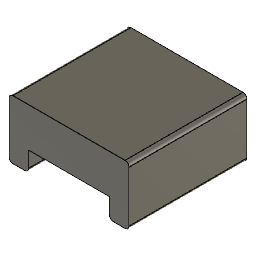
3) PLA 10mm Level Spacer (Autodesk Fusion 360 design; units mm, degrees)
Autodesk Fusion 360 part; units mm, degrees
sketch "Sketch1" plane through (0, 0, 0) normal (0, 0, 1) x (1, 0, 0)
  line L0 (10.25, 15) -> (-10.25, 15)
  line L1 (-10.25, 15) -> (-10.25, -15)
  line L2 (-10.25, -15) -> (10.25, -15)
  line L3 (10.25, -15) -> (10.25, 15)
  line L4 (10.25, 15) -> (-10.25, -15) construction
  line L5 (-10.25, 15) -> (10.25, -15) construction
  line L6 (-10.25, 15) -> (-15.25, 15)
  line L7 (-15.25, 15) -> (-15.25, -15)
  line L8 (-15.25, -15) -> (-10.25, -15)
  line L9 (-10.25, -15) -> (-10.25, 15)
  line L10 (10.25, 15) -> (15.25, 15)
  line L11 (15.25, 15) -> (15.25, -15)
  line L12 (15.25, -15) -> (10.25, -15)
  line L13 (10.25, -15) -> (10.25, 15)
  dimension "d1" = 20.5
  dimension "d2" = 30
  dimension "d3" = 5
  dimension "d4" = 30
  dimension "d5" = 5
  dimension "d6" = 30
  constraint horizontal L0
  constraint perpendicular L0 L1
  constraint parallel L0 L2
  constraint parallel L1 L3
  constraint coincident L4 origin
  constraint coincident L5 origin
  constraint horizontal L6
  constraint vertical L7
  constraint horizontal L8
  constraint vertical L9
  constraint horizontal L10
  constraint vertical L11
  constraint horizontal L12
  constraint vertical L13
  measures "d1" distance of L1.end L2.end
  measures "d2" distance of L0.end L1.end
  measures "d3" distance of L0.end L6.end
  measures "d4" distance of L0.end L1.end
  measures "d5" distance of L0.start L10.end
  measures "d6" distance of L0.start L2.end
extrude "Extrude1" add sketch "Sketch1" along normal blind 10
extrude "Extrude2" add sketch "Sketch1" against normal blind 5 contours L3 L10 L11 L12 L13 | L1 L6 L7 L8 L9
fillet "Fillet1" radius 1 6 edges at (-10.25, 0, -5) (10.25, 0, -5) (15.25, 0, -5) (-15.25, 0, -5) (-15.25, 0, 10) (15.25, 0, 10)
named bodies: "Stinger Spacer 10mm"
